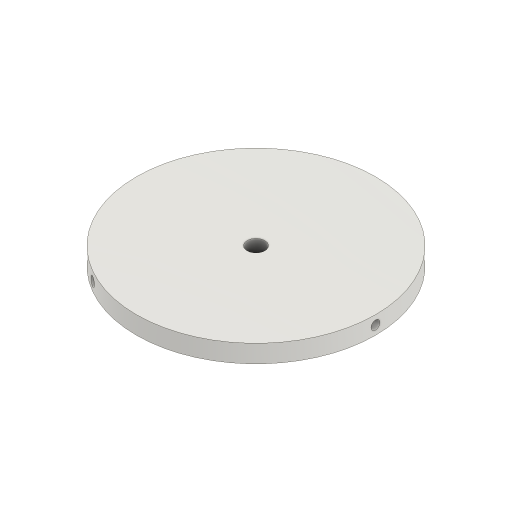
# Autodesk Inventor part: Engine bulkhead
Saved by Autodesk Inventor 2024 (Build 280153000, 153)
## iProperties
Created: 2023-12-30
Part Number: Engine bulkhead
Material: Steel AISI 1006 85 HR
Document SubType Name: Modeling
Designer: Jamie
Density: 7.872 g/cm^3
Appearance: Steel
Author: Jamie
Autodesk Inventor part; units mm, degrees
ref_plane "XZ Plane" through (0, 0, 0) normal (0, 1, 0) x (-1, 0, 0)
ref_plane "XY Plane" through (0, 0, 0) normal (0, 0, 1) x (1, 0, 0)
sketch "Sketch1" plane through (0, 0, 0) normal (0, 1, 0) x (-1, 0, 0)
  circle A0 centre (0, 0) radius 33.5
  dimension "d0" = 67
  constraints: 1 centre point, 1 coincident
  measures "d0" diameter of A0
extrude "Extrusion1" add sketch "Sketch1" along normal blind 5
ref_plane "Work Plane1" through (33.5, 0, 0) normal (1, 0, 0) x (0, 1, 0)
sketch "Sketch3" plane through (0, 0, 0) normal (0, -1, 0) x (1, 0, 0)
  point P0 (0, 0)
  point P1 (0, 0)
  constraints: 1 coincident
hole "Hole2" at (0, 0, 0) direction (0, 1, 0) diameter 5 depth 8 tip angle 118
sketch "Sketch6" plane through (33.5, 0, 0) normal (1, 0, 0) x (0, 1, 0)
  line L0 (0, -33.5) -> (0, 33.5) projected
  point P0 (0, 0)
  point P1 (2.5, 0)
  dimension "d47" = 2.5
  measures "d47" distance from line of L0 point (2.5, 0)
hole "Hole4" at (33.5, 2.5, 0) direction (-1, 0, 0) diameter 2.5 depth 10 tip angle 118
pattern_circular "Circular Pattern3" count 3 over 360 about axis through (0, 0, 0) along (0, 1, 0) of "Hole4"
body "Solid1"
